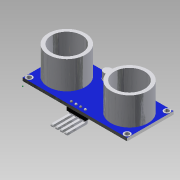
# Autodesk Inventor part: PARTE 1
Saved by Autodesk Inventor 2016 (Build 200138000, 138)
## iProperties
Created: 2016-07-30
Part Number: PARTE 1
Material: Generic
Document SubType Name: Modeling
Designer: julianesteban
Density: 1 g/cm^3
Appearance: Default
Author: julianesteban
Autodesk Inventor part; units mm, degrees
ref_plane "YZ Plane" through (0, 0, 0) normal (1, 0, 0) x (0, 1, 0)
ref_plane "XZ Plane" through (0, 0, 0) normal (0, 1, 0) x (-1, 0, 0)
ref_plane "XY Plane" through (0, 0, 0) normal (0, 0, 1) x (1, 0, 0)
sketch "Sketch1" plane through (0, 0, 0) normal (0, 0, 1) x (1, 0, 0)
  line L0 (0, 0) -> (45, 0)
  line L1 (45, 0) -> (45, 20)
  line L2 (45, 20) -> (0, 20)
  line L3 (0, 20) -> (0, 0)
  line L4 (0, 0) -> (45, 0)
  line L5 (45, 0) -> (45, 20)
  dimension "d0" = 45
  dimension "d1" = 20
  constraints: 12 end point, 2 horizontal, 2 parallel, 1 perpendicular, 1 vertical
  measures "d0" distance of L0.start L0.end
  measures "d1" distance of L0.end L1.end
extrude "Extrusion1" add sketch "Sketch1" along normal blind 1.3
sketch "Sketch2" plane through (0, 0, 1.3) normal (0, 0, 1) x (1, 0, 0)
  line L0 (0, 20) -> (0, 0)
  line L1 (0, 20) -> (0, 0) projected
  circle A0 centre (9, 10) radius 8
  line L2 (0, 0) -> (45, 0) projected
  line L3 (22.5, 0) -> (22.5, 16.923)
  circle A1 centre (36, 10) radius 8
  constraints: 4 end point, 2 centre point, 2 vertical, 1 midpoint, 1 symmetric about line, 1 other
extrude "Extrusion2" add sketch "Sketch2" along normal blind 7
sketch "Sketch3" plane through (0, 0, 1.3) normal (0, 0, 1) x (1, 0, 0)
  line L0 (0, 0) -> (45, 0) projected
  line L1 (22.5, 0) -> (22.5, 3.8703)
  line L2 (22.5, 0) -> (22.5, 1.5)
  circle A0 centre (23.5, 1.5) radius 0.5
  circle A1 centre (25.5, 1.5) radius 0.5
  circle A2 centre (21.5, 1.5) radius 0.5
  circle A3 centre (19.5, 1.5) radius 0.5
  constraints: 4 centre point, 4 end point, 2 symmetric about line, 1 midpoint, 1 point on line, 1 vertical, 2 other
extrude "Extrusion3" cut sketch "Sketch3" against normal blind 7
sketch "Sketch4" plane through (0, 0, 1.3) normal (0, 0, 1) x (1, 0, 0)
  line L0 (0, 0) -> (0.5, 0)
  line L1 (0, 0) -> (45, 0) projected
  line L2 (0.5, 0) -> (0.5, 0.5)
  circle A0 centre (1.4, 1.4) radius 0.9
  line L3 (0, 20) -> (0, 0) projected
  line L4 (0, 20) -> (0, 0) projected
  line L5 (45, 20) -> (0, 20) projected
  line L6 (0, 20) -> (0.5, 20)
  line L7 (0.5, 20) -> (0.5, 19.5)
  circle A1 centre (1.4, 18.6) radius 0.9
  line L8 (45, 0) -> (44.5, 0)
  line L9 (44.5, 0) -> (44.5, 0.5)
  circle A2 centre (43.6, 1.4) radius 0.9
  line L10 (45, 20) -> (45, 0)
  line L11 (45, 20) -> (45, 0)
  line L12 (45, 20) -> (44.5, 20)
  line L13 (44.5, 20) -> (44.5, 19.5)
  circle A3 centre (43.6, 18.6) radius 0.9
  constraints: 20 end point, 4 centre point, 1 point on line, 1 vertical
extrude "Extrusion4" cut sketch "Sketch4" against normal blind 7 contours A0 | A1 | A2 | A3
sketch "Sketch5" plane through (9, 10, 8.3) normal (0, 0, 1) x (1, 0, 0)
  circle A0 centre (27, 0) radius 8 projected
  circle A1 centre (0, 0) radius 8 projected
  circle A2 centre (0, 0) radius 6.5
  circle A3 centre (27, 0) radius 6.5
  point P0 (-9, -10)
  dimension "d21" = 13
  dimension "d22" = 13
  constraints: 2 centre point, 2 coincident
  measures "d21" diameter of A2
  measures "d22" diameter of A3
extrude "Extrusion5" cut sketch "Sketch5" against normal blind 10 contours A2 | A3
sketch "Sketch6" plane through (9, 10, 8.3) normal (0, 0, 1) x (1, 0, 0)
  circle A0 centre (27, 0) radius 6.5 projected
  circle A1 centre (27, 0) radius 8 projected
  circle A2 centre (0, 0) radius 6.5 projected
  circle A3 centre (0, 0) radius 8 projected
  point P0 (-9, -10)
extrude "Extrusion6" add sketch "Sketch6" along normal blind 5
sketch "Sketch7" plane through (0, 0, 0) normal (0, 0, -1) x (-1, 0, 0)
  circle A0 centre (-36, 10) radius 6.5 projected
  circle A1 centre (-9, 10) radius 6.5 projected
  circle A2 centre (-43.6, 1.4) radius 0.9 projected
  circle A3 centre (-1.4, 1.4) radius 0.9 projected
  circle A4 centre (-1.4, 18.6) radius 0.9 projected
  circle A5 centre (-43.6, 18.6) radius 0.9 projected
  circle A6 centre (-21.5, 1.5) radius 0.5 projected
  circle A7 centre (-23.5, 1.5) radius 0.5 projected
  circle A8 centre (-25.5, 1.5) radius 0.5 projected
  circle A9 centre (-19.5, 1.5) radius 0.5 projected
  line L0 (0, 0) -> (-45, 0) projected
  line L1 (0, 20) -> (0, 0) projected
  line L2 (-45, 20) -> (0, 20) projected
  line L3 (-45, 0) -> (-45, 20) projected
extrude "Extrusion7" add sketch "Sketch7" against normal blind 1 contours A0 | A1
sketch "Sketch8" plane through (0, 0, 1.3) normal (0, 0, 1) x (1, 0, 0)
  circle A0 centre (43.6, 1.4) radius 0.9 projected
  circle A1 centre (1.4, 1.4) radius 0.9 projected
  circle A2 centre (1.4, 18.6) radius 0.9 projected
  circle A3 centre (43.6, 18.6) radius 0.9 projected
  circle A4 centre (21.5, 1.5) radius 0.5 projected
  circle A5 centre (23.5, 1.5) radius 0.5 projected
  circle A6 centre (25.5, 1.5) radius 0.5 projected
  circle A7 centre (19.5, 1.5) radius 0.5 projected
  circle A8 centre (9, 10) radius 8 projected
  circle A9 centre (36, 10) radius 8 projected
  line L0 (0, 0) -> (45, 0) projected
  line L1 (45, 0) -> (45, 20) projected
  line L2 (45, 20) -> (0, 20) projected
  line L3 (0, 20) -> (0, 0) projected
  line L4 (45, 20) -> (0, 20) projected
  line L5 (22.5, 20) -> (28, 20)
  line L6 (28, 20) -> (17, 20)
  line L7 (22.5, 20) -> (22.5, 19.5)
  line L8 (22.5, 19.5) -> (26.25, 19.5)
  line L9 (18.75, 16) -> (26.25, 16)
  arc A10 (26.25, 16) -> (26.25, 19.5) centre (26.25, 17.75) ccw
  line L10 (22.5, 19.5) -> (18.75, 19.5)
  arc A11 (18.75, 19.5) -> (18.75, 16) centre (18.75, 17.75) ccw
  line L11 (26.25, 19.5) -> (18.75, 19.5)
  line L12 (17, 19.5) -> (16.3922, 19.5)
  constraints: 16 end point, 4 point on circle, 3 symmetric about line, 2 centre point, 2 horizontal, 2 parallel, 2 point on line, 1 midpoint, 1 perpendicular, 1 vertical, 1 other
extrude "Extrusion8" add sketch "Sketch8" along normal blind 0.2 contours L8 A10 L9 A11 L10
sketch "Sketch9" plane through (0, 0, 1.5) normal (0, 0, 1) x (1, 0, 0)
  line L0 (26.25, 19.5) -> (18.75, 19.5) projected
  arc A0 (18.75, 19.5) -> (18.75, 16) centre (18.75, 17.75) ccw projected
  line L1 (18.75, 16) -> (26.25, 16) projected
  arc A1 (26.25, 16) -> (26.25, 19.5) centre (26.25, 17.75) ccw projected
  line L2 (26.25, 19.5) -> (18.75, 19.5) projected
  line L3 (22.5, 19.5) -> (22.5, 19.4)
  line L4 (22.5, 19.4) -> (26.25, 19.4)
  line L5 (22.5, 19.4) -> (18.75, 19.4)
  line L6 (18.75, 16) -> (18.75, 16.1)
  line L7 (18.75, 16) -> (18.85, 16) construction
  line L8 (18.75, 16.1) -> (26.25, 16.1)
  arc A2 (18.75, 19.4) -> (18.75, 16.1) centre (18.75, 17.75) ccw
  arc A3 (26.25, 16.1) -> (26.25, 19.4) centre (26.25, 17.75) ccw
  point P0 (0, 0)
  constraints: 12 end point, 4 point on circle, 2 centre point, 2 coincident, 2 horizontal, 2 perpendicular, 2 vertical, 1 midpoint, 1 point on line, 1 tangent
extrude "Extrusion9" add sketch "Sketch9" along normal blind 3 contours L4 A3 L8 A2 L5
sketch "Sketch10" plane through (0, 0, 1.3) normal (0, 0, 1) x (1, 0, 0)
  circle A0 centre (1.4, 18.6) radius 0.9 projected
  circle A1 centre (1.4, 18.6) radius 1.35
  arc A2 (26.25, 16) -> (26.25, 19.5) centre (26.25, 17.75) ccw projected
  line L0 (26.25, 16) -> (18.75, 16) projected
  arc A3 (18.75, 19.5) -> (18.75, 16) centre (18.75, 17.75) ccw projected
  line L1 (18.75, 19.5) -> (26.25, 19.5) projected
  circle A4 centre (43.6, 1.4) radius 0.9 projected
  circle A5 centre (1.4, 1.4) radius 0.9 projected
  circle A6 centre (1.4, 18.6) radius 0.9 projected
  circle A7 centre (43.6, 18.6) radius 0.9 projected
  circle A8 centre (21.5, 1.5) radius 0.5 projected
  circle A9 centre (23.5, 1.5) radius 0.5 projected
  circle A10 centre (25.5, 1.5) radius 0.5 projected
  circle A11 centre (19.5, 1.5) radius 0.5 projected
  circle A12 centre (9, 10) radius 8 projected
  circle A13 centre (36, 10) radius 8 projected
  line L2 (0, 0) -> (45, 0) projected
  line L3 (45, 0) -> (45, 20) projected
  line L4 (45, 20) -> (0, 20) projected
  line L5 (0, 20) -> (0, 0) projected
  circle A14 centre (1.4, 1.4) radius 1.35
  circle A15 centre (43.6, 1.4) radius 1
  circle A16 centre (43.6, 18.6) radius 1.35
  dimension "d44" = 2.7
  dimension "d45" = 2.7
  dimension "d46" = 2
  dimension "d47" = 2.7
  constraints: 4 centre point, 4 coincident
  measures "d44" diameter of A1
  measures "d45" diameter of A14
  measures "d46" diameter of A15
  measures "d47" diameter of A16
extrude "Extrusion10" add sketch "Sketch10" along normal blind 0.1 contours A1 | A14 | A16
sketch "Sketch11" plane through (0, 0, 1.3) normal (0, 0, 1) x (1, 0, 0)
  circle A0 centre (43.6, 1.4) radius 0.9 projected
  circle A1 centre (43.6, 1.4) radius 1.35
  point P0 (0, 0)
  dimension "d50" = 2.7
  constraints: 1 centre point, 1 coincident
  measures "d50" diameter of A1
extrude "Extrusion11" add sketch "Sketch11" along normal blind 0.1
sketch "Sketch12" plane through (0, 0, 1.3) normal (0, 0, 1) x (1, 0, 0)
  circle A0 centre (19.5, 1.5) radius 0.5 projected
  circle A1 centre (21.5, 1.5) radius 0.5 projected
  circle A2 centre (23.5, 1.5) radius 0.5 projected
  circle A3 centre (25.5, 1.5) radius 0.5 projected
  line L0 (19.5, 0.8729) -> (19.5, 2)
  line L1 (21.5, 1) -> (21.5, 2)
  line L2 (23.5, 1) -> (23.5, 2)
  line L3 (25.5, 1) -> (25.5, 2)
  circle A4 centre (25.5, 1.5) radius 0.5 projected
  circle A5 centre (25.5, 1.5) radius 0.5 projected
  point P0 (0, 0)
  constraints: 8 end point, 6 point on circle, 2 parallel, 1 vertical, 1 vertical alignment, 1 other
revolve "Revolution1" add sketch "Sketch12" angle 360 about axis through (21.5, 1, 1.3) along (0, 1, 0) picked at (21.3442, 1.4409) contours L1 A1
sketch "Sketch13" plane through (0, 0, 1.3) normal (0, 0, 1) x (1, 0, 0)
  circle A0 centre (43.6, 1.4) radius 1.35 projected
  circle A1 centre (43.6, 18.6) radius 1.35 projected
  circle A2 centre (1.4, 18.6) radius 1.35 projected
  circle A3 centre (1.4, 1.4) radius 1.35 projected
  arc A4 (26.25, 16) -> (26.25, 19.5) centre (26.25, 17.75) ccw projected
  line L0 (26.25, 16) -> (18.75, 16) projected
  arc A5 (18.75, 19.5) -> (18.75, 16) centre (18.75, 17.75) ccw projected
  line L1 (18.75, 19.5) -> (26.25, 19.5) projected
  circle A6 centre (21.5, 1.5) radius 0.5 projected
  circle A7 centre (23.5, 1.5) radius 0.5 projected
  circle A8 centre (25.5, 1.5) radius 0.5 projected
  circle A9 centre (19.5, 1.5) radius 0.5 projected
  circle A10 centre (9, 10) radius 8 projected
  circle A11 centre (36, 10) radius 8 projected
  line L2 (0, 0) -> (45, 0) projected
  line L3 (45, 0) -> (45, 20) projected
  line L4 (45, 20) -> (0, 20) projected
  line L5 (0, 20) -> (0, 0) projected
  circle A12 centre (23.5, 1.5) radius 0.5 projected
  line L6 (23.5, 1.5) -> (23.5, 1)
  line L7 (23.5, 1.5) -> (24, 1.5) construction
  line L8 (23.5, 1) -> (23.5, 2.2277)
  line L9 (25.5, 1.5) -> (25.5, 2)
  line L10 (19.5, 1.1367) -> (19.5, 2.962)
  line L11 (19.5, 2.962) -> (19.5, 0.5552)
  circle A13 centre (19.5, 1.5) radius 0.5 projected
  arc A14 (19.5, 2) -> (19.5, 1) centre (19.5, 1.5) ccw
  dimension "d54" = 90
  constraints: 12 end point, 4 point on circle, 4 point on line, 2 vertical, 2 vertical alignment, 1 centre point, 1 horizontal, 1 perpendicular, 2 other
  measures "d54" angle of L6 L7
revolve "Revolution2" add sketch "Sketch13" angle 360 about axis through (19.5, 2.962, 1.3) along (0, -1, 0) picked at (19.4601, 1.7074) contours L10 L11 A9
sketch "Sketch14" plane through (0, 0, 1.3) normal (0, 0, 1) x (1, 0, 0)
  circle A0 centre (23.5, 1.5) radius 0.5 projected
  line L0 (23.5, 0.6366) -> (23.5, 2.6305)
  arc A1 (23.5, 2) -> (23.5, 1) centre (23.5, 1.5) ccw
  point P0 (0, 0)
  constraints: 4 point on circle, 2 end point, 2 point on line, 1 centre point, 1 concentric, 1 vertical
revolve "Revolution3" add sketch "Sketch14" angle 360 about axis through (23.5, 0.6366, 1.3) along (0, 1, 0) picked at (23.3442, 1.4409) contours L0 A0
sketch "Sketch15" plane through (0, 0, 1.3) normal (0, 0, 1) x (1, 0, 0)
  line L0 (25.5, 1) -> (25.5, 2)
  arc A0 (25.5, 2) -> (25.5, 1) centre (25.5, 1.5) ccw
  point P0 (0, 0)
  constraints: 2 end point, 2 point on circle, 1 centre point, 1 vertical
revolve "Revolution4" add sketch "Sketch15" angle 360 about axis through (25.5, 1, 1.3) along (0, 1, 0)
sketch "Sketch16" plane through (0, 0, 0) normal (0, 0, -1) x (-1, 0, 0)
  circle A0 centre (-43.6, 1.4) radius 0.9 projected
  circle A1 centre (-1.4, 1.4) radius 0.9 projected
  circle A2 centre (-1.4, 18.6) radius 0.9 projected
  circle A3 centre (-43.6, 18.6) radius 0.9 projected
  circle A4 centre (-21.5, 1.5) radius 0.5 projected
  circle A5 centre (-23.5, 1.5) radius 0.5 projected
  circle A6 centre (-25.5, 1.5) radius 0.5 projected
  circle A7 centre (-19.5, 1.5) radius 0.5 projected
  line L0 (0, 0) -> (-45, 0) projected
  line L1 (0, 20) -> (0, 0) projected
  line L2 (-45, 20) -> (0, 20) projected
  line L3 (-45, 0) -> (-45, 20) projected
  line L4 (-18.5, 2.5) -> (-20.5, 2.5)
  line L5 (-20.5, 2.5) -> (-20.5, 0.5)
  line L6 (-20.5, 0.5) -> (-18.5, 0.5)
  line L7 (-18.5, 0.5) -> (-18.5, 2.5)
  line L8 (-18.5, 2.5) -> (-20.5, 0.5) construction
  line L9 (-20.5, 2.5) -> (-18.5, 0.5) construction
  line L10 (-24.5, 2.5) -> (-26.5, 2.5)
  line L11 (-26.5, 2.5) -> (-26.5, 0.5)
  line L12 (-26.5, 0.5) -> (-24.5, 0.5)
  line L13 (-24.5, 0.5) -> (-24.5, 2.5)
  line L14 (-24.5, 2.5) -> (-26.5, 0.5) construction
  line L15 (-26.5, 2.5) -> (-24.5, 0.5) construction
  line L16 (-18.5, 0.5) -> (-26.5917, 0.5)
  line L17 (-18.5, 2.5917) -> (-18.5, 0.5)
  line L18 (-26.5917, 0.5) -> (-18.5, 0.5)
  line L19 (-18.5, 0.5) -> (-18.5, 2.5917)
  line L20 (-18.5, 0.5) -> (-26.5, 0.5)
  line L21 (-26.5, 0.5) -> (-26.5, 2.5)
  line L22 (-26.5, 2.5) -> (-18.5, 2.5)
  line L23 (-18.5, 2.5) -> (-18.5, 0.5)
  dimension "d58" = 2
  dimension "d59" = 2
  dimension "d60" = 2
  dimension "d61" = 2
  constraints: 40 end point, 6 parallel, 4 horizontal, 4 midpoint, 3 perpendicular
  measures "d58" distance of L6.end L5.end
  measures "d59" distance of L5.end L4.end
  measures "d60" distance of L12.end L11.end
  measures "d61" distance of L11.end L10.end
extrude "Extrusion12" add sketch "Sketch16" along normal blind 2 contours A4 | A5 | A6 | A7 | L7 L6 L5 L4 | L5 L16 L13 L22 | L13 L12 L11 L10
sketch "Sketch17" plane through (0, 0, -2) normal (0, 0, -1) x (-1, 0, 0)
  point P0 (0, 0)
sketch "Sketch18" plane through (0, 0, -2) normal (0, 0, -1) x (-1, 0, 0)
  point P0 (0, 0)
sketch "Sketch19" plane through (0, 0, -2) normal (0, 0, -1) x (-1, 0, 0)
  line L0 (-26.5, 2.5) -> (-26.5, 0.5) projected
  line L1 (-26.5, 0.5) -> (-18.5, 0.5) projected
  line L2 (-18.5, 0.5) -> (-18.5, 2.5) projected
  line L3 (-18.5, 2.5) -> (-26.5, 2.5) projected
  circle A0 centre (-19.5, 1.5) radius 0.5 projected
  circle A1 centre (-21.5, 1.5) radius 0.5 projected
  circle A2 centre (-23.5, 1.5) radius 0.5 projected
  circle A3 centre (-25.5, 1.5) radius 0.5 projected
  line L4 (-19, 2) -> (-20, 2)
  line L5 (-20, 2) -> (-20, 1)
  line L6 (-20, 1) -> (-19, 1)
  line L7 (-19, 1) -> (-19, 2)
  line L8 (-19, 2) -> (-20, 1) construction
  line L9 (-20, 2) -> (-19, 1) construction
  line L10 (-21, 2) -> (-22, 2)
  line L11 (-22, 2) -> (-22, 1)
  line L12 (-22, 1) -> (-21, 1)
  line L13 (-21, 1) -> (-21, 2)
  line L14 (-21, 2) -> (-22, 1) construction
  line L15 (-22, 2) -> (-21, 1) construction
  line L16 (-23, 2) -> (-24, 2)
  line L17 (-24, 2) -> (-24, 1)
  line L18 (-24, 1) -> (-23, 1)
  line L19 (-23, 1) -> (-23, 2)
  line L20 (-23, 2) -> (-24, 1) construction
  line L21 (-24, 2) -> (-23, 1) construction
  line L22 (-25, 2) -> (-26, 2)
  line L23 (-26, 2) -> (-26, 1)
  line L24 (-26, 1) -> (-25, 1)
  line L25 (-25, 1) -> (-25, 2)
  line L26 (-25, 2) -> (-26, 1) construction
  line L27 (-26, 2) -> (-25, 1) construction
  point P0 (0, 0)
  constraints: 48 end point, 8 midpoint, 8 parallel, 4 horizontal, 4 perpendicular, 3 point on line
extrude "Extrusion13" add sketch "Sketch19" along normal blind 2 contours A0 | L7 L6 A0 | A0 L4 L7 | A0 L5 L4 | L6 L5 A0 | A1 | L13 L12 A1 | A1 L10 L13 | A1 L11 L10 | L12 L11 A1 | A2 | L19 L18 A2 | A2 L16 L19 | A2 L17 L16 | L18 L17 A2 | A3 | L25 L24 A3 | A3 L22 L25 | A3 L23 L22 | L24 L23 A3
sketch "Sketch20" plane through (25, 1, -2) normal (0, -1, 0) x (1, 0, 0)
  line L0 (-2, 0) -> (-1, 0) projected
  line L1 (-2, 0) -> (-2, -2) projected
  line L2 (-1, -2) -> (-2, -2) projected
  line L3 (-1, 0) -> (-1, -2) projected
  line L4 (-4, 0) -> (-4, -2) projected
  line L5 (-4, 0) -> (-3, 0) projected
  line L6 (-4, 0) -> (-4, -2) projected
  line L7 (-3, -2) -> (-4, -2) projected
  line L8 (-3, 0) -> (-3, -2) projected
  line L9 (-6, 0) -> (-5, 0) projected
  line L10 (-6, 0) -> (-6, -2) projected
  line L11 (-5, -2) -> (-6, -2) projected
  line L12 (-5, 0) -> (-5, -2) projected
  line L13 (-5, 0) -> (-5, -2) projected
  line L14 (-6, -2) -> (-5, -2)
  line L15 (-5, -2) -> (-5, -1)
  line L16 (-5, -1) -> (-6, -1)
  line L17 (-6, -1) -> (-6, -2)
  line L18 (-4, -2) -> (-3, -2)
  line L19 (-3, -2) -> (-3, -1)
  line L20 (-3, -1) -> (-4, -1)
  line L21 (-4, -1) -> (-4, -2)
  line L22 (-1, 0) -> (-1, -2) projected
  line L23 (-2, -2) -> (-1, -2)
  line L24 (-1, -2) -> (-1, -1)
  line L25 (-1, -1) -> (-2, -1)
  line L26 (-2, -1) -> (-2, -2)
  line L27 (1, 0) -> (1, -2) projected
  line L28 (0, -2) -> (1, -2)
  line L29 (1, -2) -> (1, -1)
  line L30 (1, -1) -> (0, -1)
  line L31 (0, -1) -> (0, -2)
  point P0 (-25, 2)
  constraints: 32 end point, 8 parallel, 4 horizontal, 4 midpoint, 4 perpendicular
extrude "Extrusion14" add sketch "Sketch20" along normal blind 8 contours L25 L3 L2 L1 | L20 L8 L7 L4 | L16 L12 L11 L10 | L27 L28 L31 L30
sketch "Sketch21" plane through (26, 1, -2) normal (1, 0, 0) x (0, 0, -1)
  line L0 (0, 0) -> (0, 1) projected
  line L1 (0, 0) -> (1, 0) projected
  line L2 (1, 0) -> (1, -8) projected
  line L3 (2, -8) -> (1, -8) projected
  line L4 (2, 1) -> (2, -8) projected
  line L5 (0, 1) -> (2, 1) projected
  line L6 (2, 1) -> (2, -8) projected
  line L7 (0, 1) -> (2, 1) projected
  arc A0 (2, 0.6759) -> (1.5939, 1) centre (1.5412, 0.5175) ccw
  line L8 (1, 0) -> (1, -8) projected
  line L9 (0, 0) -> (1, 0) projected
  line L10 (2, -8) -> (1, -8) projected
  line L11 (1.5, -8) -> (2, -8)
  line L12 (1.5, -8) -> (1.5, -7.5)
  arc A1 (1, -7.5) -> (2, -7.5) centre (1.5, -7.5) ccw
  point P0 (-2, -1)
  dimension "d68" = 0.5
  dimension "d69" = 0.5
  constraints: 5 point on circle, 4 end point, 4 point on line, 2 centre point, 1 coincident, 1 collinear, 1 midpoint, 1 vertical
  measures "d68" distance of L11.start L3.start
  measures "d69" distance of L11.start L12.end
extrude "Extrusion15" cut sketch "Sketch21" against normal blind 80 contours L5 L4 A0 | A1 L3 L2 | A1 L4 L3
body "Solid1"
